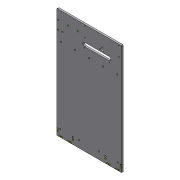
# Autodesk Inventor part: TL20240901-10320CV-002
Saved by Autodesk Inventor 2022.5 (Build 265521000, 521)
## iProperties
Category: FOLLOWER UNIT ASSY
Manager: 호상태
Company: 현대 트랜시스
RuleStatus: InUse
Created: 2023-01-19
Part Number: TL20240901-10320CV-002
Project: MEa-PJT 2LINE
Checked By: 김형민
Engr Approved By: 김형민
User Status: 1/1 x6
Material: SS400
Description: 0
Document SubType Name: Modeling
Mfg Approved By: 호상태
Designer: 박성규
Stock Number: 002
Mass: 13148.3 g
Surface Area: 1560.92 cm^2
Volume: 1670.68 cm^3
Density: 7.85 g/cm^3
Appearance: Painting-RAL7035
BeforeDocSave0: file://Part Design STD iLogic
DETAIL: Coveryor Assembly
M/C TITLE: MEa/NEa차종 시트조립라인
SPECIFICATION: TL20221201-000000CV-005
DocNumber: 221118_Standard_v1
Folder: .\
VDS_Category: 엔지니어링
Detail Description: Processed products
Title: SIDE PLATE
Subject: MEa차종 시트조립2라인
Author: 박성규
Revision Number: A
Autodesk Inventor part; units mm, degrees
ref_plane "YZ Plane" through (0, 0, 0) normal (1, 0, 0) x (0, 1, 0)
ref_plane "XZ Plane" through (0, 0, 0) normal (0, 1, 0) x (-1, 0, 0)
ref_plane "XY Plane" through (0, 0, 0) normal (0, 0, 1) x (1, 0, 0)
sketch "스케치22" plane through (0, 0, 0) normal (0, 0, 1) x (1, 0, 0)
  line L0 (-230, 390) -> (230, 390)
  line L1 (230, 390) -> (230, -390)
  line L2 (230, -390) -> (-230, -390)
  line L3 (-230, -390) -> (-230, 390)
  line L4 (-230, 390) -> (230, -390) construction
  line L5 (230, 390) -> (-230, -390) construction
  point P0 (0, 0)
  dimension "d122" = 460
  dimension "HIGHT" = 780
  constraints: 12 end point, 2 midpoint, 2 parallel, 1 horizontal, 1 perpendicular
  measures "d122" distance of L0.start L0.end
  measures "HIGHT" distance of L0.end L1.end
extrude "돌출12" add sketch "스케치22" along normal blind 12
sketch "스케치23" plane through (0, 0, 12) normal (0, 0, 1) x (1, 0, 0)
  line L0 (230, 390) -> (-230, 390) construction
  line L1 (-230, 390) -> (-230, -390) construction
  point P0 (0, 0)
  point P1 (-220, 324)
  point P2 (-220, 264)
  point P3 (-190, 264)
  point P4 (-150, 324)
  point P5 (-80, 324)
  point P6 (-220, -246)
  point P7 (-150, -246)
  point P8 (-80, -246)
  point P9 (-220, -306)
  point P10 (-190, -306)
  dimension "d126" = 66
  dimension "d128" = 126
  dimension "d129" = 10
  dimension "d130" = 10
  dimension "d131" = 70
  dimension "d132" = 70
  dimension "d133" = 30
  dimension "d154" = 10
  dimension "d155" = 30
  dimension "d156" = 696
  dimension "d157" = 636
  dimension "d158" = 10
  dimension "d159" = 70
  dimension "d160" = 70
  constraints: 6 horizontal alignment
  measures "d126" distance from line of L0 point (-220, 324)
  measures "d128" distance from line of L0 point (-220, 264)
  measures "d129" distance from line of L1 point (-220, 324)
  measures "d130" distance from line of L1 point (-220, 264)
  measures "d131" distance of point (-150, 324) point (-220, 324)
  measures "d132" distance of point (-80, 324) point (-150, 324)
  measures "d133" distance of point (-190, 264) point (-220, 264)
  measures "d154" distance from line of L1 point (-220, -306)
  measures "d155" distance of point (-220, -306) point (-190, -306)
  measures "d156" distance from line of L0 point (-220, -306)
  measures "d157" distance from line of L0 point (-220, -246)
  measures "d158" distance from line of L1 point (-220, -246)
  measures "d159" distance of point (-150, -246) point (-220, -246)
  measures "d160" distance of point (-80, -246) point (-150, -246)
hole "구멍7" at (-220, 324, 12) at (-220, 264, 12) at (-190, 264, 12) at (-150, 324, 12) at (-80, 324, 12) direction (0, 0, -1) diameter 9 end through all clearance for "Socket Head Cap Screw" size "M8" standard "TS Profile"
sketch "스케치24" plane through (0, 0, 12) normal (0, 0, 1) x (1, 0, 0)
  line L0 (230, 390) -> (-230, 390) construction
  line L1 (-230, 390) -> (-230, -390) construction
  line L2 (230, -390) -> (230, 390) construction
  line L3 (-230, -390) -> (230, -390) projected
  point P0 (0, 0)
  point P1 (-200, 198)
  point P2 (-100, 198)
  point P3 (0, 198)
  point P4 (100, 198)
  point P5 (200, 198)
  point P6 (55, -372)
  point P7 (0, -372)
  point P8 (-55, -372)
  point P9 (-110, -372)
  point P10 (110, -372)
  dimension "d141" = 30
  dimension "d142" = 192
  dimension "d143" = 100
  dimension "d144" = 100
  dimension "d145" = 100
  dimension "d146" = 100
  dimension "d231" = 55
  dimension "d234" = 120
  dimension "d308" = 120
  dimension "d338" = 18
  dimension "d339" = 55
  dimension "d340" = 55
  dimension "d341" = 55
  constraints: 8 horizontal alignment
  measures "d141" distance from line of L1 point (-200, 198)
  measures "d142" distance from line of L0 point (-200, 198)
  measures "d143" distance of point (-100, 198) point (-200, 198)
  measures "d144" distance of point (0, 198) point (-100, 198)
  measures "d145" distance of point (0, 198) point (100, 198)
  measures "d146" distance of point (200, 198) point (100, 198)
  measures "d231" distance of point (-55, -372) point (-110, -372)
  measures "d234" distance from line of L1 point (-110, -372)
  measures "d308" distance from line of L2 point (110, -372)
  measures "d338" distance from line of point (-110, -372) L3
  measures "d339" distance of point (0, -372) point (55, -372)
  measures "d340" distance of point (-55, -372) point (0, -372)
  measures "d341" distance of point (55, -372) point (110, -372)
hole "구멍8" at (-200, 198, 12) at (-100, 198, 12) at (0, 198, 12) at (100, 198, 12) at (200, 198, 12) direction (0, 0, -1) diameter 9 end through all clearance for "Socket Head Cap Screw" size "M8" standard "TS Profile"
fillet "모깎기6" radius 5 2 edges at (-230, 390, 6) (230, 390, 6)
sketch "스케치29" plane through (0, 0, 12) normal (0, 0, 1) x (1, 0, 0)
  line L0 (230, -390) -> (230, 385) construction
  line L1 (225, 390) -> (-225, 390) construction
  point P0 (0, 0)
  point P1 (210, 382)
  point P2 (-30, 382)
  point P3 (210, -188)
  point P4 (-30, -188)
  dimension "d199" = 8
  dimension "d200" = 20
  dimension "d201" = 240
  dimension "d202" = 570
  constraints: 2 horizontal alignment, 2 vertical alignment
  measures "d199" distance from line of L1 point (210, 382)
  measures "d200" distance from line of L0 point (210, 382)
  measures "d201" distance of point (-30, 382) point (210, 382)
  measures "d202" distance of point (210, -188) point (210, 382)
hole "구멍11" at (210, 382, 12) at (-30, 382, 12) direction (0, 0, -1) diameter 4.917 end through all thread size "M6x1" class "6H" standard "TS profile"
sketch "스케치31" plane through (0, 0, 0) normal (0, 0, -1) x (-1, 0, 0)
  line L0 (-230, -390) -> (-230, 385) construction
  line L1 (-225, 390) -> (225, 390) construction
  point P0 (-75, 375)
  point P1 (-162, 375)
  point P2 (0, 0)
  point P3 (-210, 311)
  point P4 (-90, 311)
  point P5 (30, 311)
  point P6 (-198, 375)
  point P7 (-196, 375)
  dimension "d219" = 79
  dimension "d220" = 20
  dimension "d221" = 120
  dimension "d222" = 120
  constraints: 2 horizontal alignment, 1 other
  measures "d220" distance from line of L0 point (-210, 311)
  measures "d221" distance of point (-90, 311) point (-210, 311)
  measures "d222" distance of point (-90, 311) point (30, 311)
hole "구멍13" at (210, 311, 0) at (90, 311, 0) at (-30, 311, 0) direction (0, 0, 1) diameter 6.6 end through all clearance for "Socket Head Cap Screw" size "M6" standard "TS Profile"
sketch "스케치43" plane through (0, 0, 0) normal (0, 0, -1) x (-1, 0, 0)
  line L0 (230, 385) -> (230, -390) projected
  line L1 (230, -390) -> (-230, -390) projected
  point P0 (0, 0)
  point P1 (205, -340)
  point P2 (70, -340)
  point P3 (-70, -340)
  point P4 (-205, -340)
  dimension "d309" = 135
  dimension "d310" = 140
  dimension "d311" = 135
  dimension "d312" = 25
  dimension "d314" = 50
  constraints: 3 horizontal alignment
  measures "d309" distance of point (70, -340) point (205, -340)
  measures "d310" distance of point (-70, -340) point (70, -340)
  measures "d311" distance of point (-205, -340) point (-70, -340)
  measures "d312" distance from line of L0 point (205, -340)
  measures "d314" distance from line of L1 point (205, -340)
hole "구멍18" at (-205, -340, 0) at (-70, -340, 0) at (70, -340, 0) at (205, -340, 0) direction (0, 0, 1) diameter 9 end through all clearance for "Socket Head Cap Screw" size "M8" standard "TS Profile"
sketch "스케치44" plane through (0, 0, 12) normal (0, 0, 1) x (1, 0, 0)
  line L0 (-116, -361) -> (-224, -361)
  line L1 (-224, -361) -> (-224, -346)
  line L2 (-224, -346) -> (-116, -346)
  line L3 (-116, -346) -> (-116, -361)
  line L4 (-116, -361) -> (-224, -346) construction
  line L5 (-224, -361) -> (-116, -346) construction
  line L6 (-230, 385) -> (-230, -390) projected
  line L7 (-230, -390) -> (230, -390) projected
  point P0 (0, 0)
  point P1 (-210, -384)
  point P2 (-195, -384)
  point P3 (-145, -384)
  point P4 (-130, -384)
  point P5 (-170, -353.5)
  dimension "d322" = 108
  dimension "d323" = 15
  dimension "d324" = 20
  dimension "d325" = 15
  dimension "d326" = 50
  dimension "d327" = 15
  dimension "d328" = 6
  dimension "d329" = 29
  dimension "d330" = 6
  constraints: 12 end point, 3 horizontal alignment, 2 midpoint, 2 parallel, 1 horizontal, 1 perpendicular
  measures "d322" distance of L0.start L0.end
  measures "d323" distance of L2.end L0.start
  measures "d324" distance from line of L6 point (-210, -384)
  measures "d325" distance of point (-195, -384) point (-210, -384)
  measures "d326" distance of point (-145, -384) point (-195, -384)
  measures "d327" distance of point (-130, -384) point (-145, -384)
  measures "d328" distance between parallel lines of L6 L1
  measures "d329" distance between parallel lines of L7 L0
  measures "d330" distance from line of L7 point (-210, -384)
hole "구멍19" at (-210, -384, 12) at (-195, -384, 12) at (-145, -384, 12) at (-130, -384, 12) at (-224, -361, 12) at (-224, -346, 12) at (-116, -361, 12) at (-116, -346, 12) direction (0, 0, -1) diameter 6.6 end through all counterbore diameter 11 counterbore depth 6.5 clearance for "Socket Head Cap Screw" size "M6" standard "TS Profile"
mirror "미러2" about plane through (0, 0, 0) normal (1, 0, 0) of "구멍19"
sketch "Sketch45" plane through (0, 0, 0) normal (0, 0, -1) x (-1, 0, 0)
  line L0 (-155, 254) -> (45, 254)
  line L1 (45, 254) -> (45, 280)
  line L2 (45, 280) -> (-155, 280)
  line L3 (-155, 280) -> (-155, 254)
  line L4 (-230, -390) -> (-230, 385) projected
  line L5 (-225, 390) -> (225, 390) projected
  point P0 (0, 0)
  dimension "d342" = 200
  dimension "d343" = 26
  dimension "d344" = 75
  dimension "d345" = 110
  constraints: 8 end point, 2 parallel, 1 horizontal, 1 perpendicular
  measures "d342" distance of L2.end L1.end
  measures "d343" distance of L1.end L0.end
  measures "d344" distance between parallel lines of L4 L3
  measures "d345" distance between parallel lines of L5 L2
extrude "Extrusion22" cut sketch "Sketch45" along normal through all both and the other way through all
sketch "Sketch46" plane through (0, 0, 0) normal (0, 0, -1) x (-1, 0, 0)
  line L0 (45, 254) -> (-155, 254) projected
  line L1 (-155, 254) -> (-155, 280) projected
  line L2 (45, 280) -> (45, 254) projected
  point P0 (0, 0)
  point P1 (-145, 244.5)
  point P2 (35, 244.5)
  dimension "d348" = 9.5
  dimension "d349" = 10
  dimension "d350" = 10
  constraints: 1 horizontal alignment
  measures "d348" distance from line of point (-145, 244.5) L0
  measures "d349" distance from line of point (-145, 244.5) L1
  measures "d350" distance from line of point (35, 244.5) L2
hole "Hole20" at (145, 244.5, 0) at (-35, 244.5, 0) direction (0, 0, 1) diameter 4.134 end through all thread size "M5x0.8" class "6H" standard "TS profile"
fillet "Fillet8" radius 13 4 edges at (155, 254, 6) (155, 280, 6) (-45, 254, 6) (-45, 280, 6)
sketch "Sketch47" plane through (0, 0, 0) normal (0, 0, -1) x (-1, 0, 0)
  line L0 (-80, 294.35) -> (-100, 294.35) construction
  line L1 (-80, 299.35) -> (-100, 299.35)
  line L2 (-100, 289.35) -> (-80, 289.35)
  arc A0 (-80, 289.35) -> (-80, 299.35) centre (-80, 294.35) ccw
  arc A1 (-100, 299.35) -> (-100, 289.35) centre (-100, 294.35) ccw
  line L3 (-230, -390) -> (-230, 385) projected
  line L4 (-225, 390) -> (225, 390) projected
  point P0 (0, 0)
  point P1 (-90, 294.35)
  dimension "d359" = 10
  dimension "d360" = 10
  dimension "d361" = 140
  dimension "d362" = 95.65
  constraints: 8 end point, 4 point on circle, 4 tangent, 2 centre point, 1 horizontal, 1 midpoint, 1 parallel
  measures "d359" distance of point (-90, 294.35) L0.end
  measures "d360" diameter of A1
  measures "d361" distance from line of point (-90, 294.35) L3
  measures "d362" distance between parallel lines of L4 L0
extrude "Extrusion23" cut sketch "Sketch47" along normal through all both and the other way through all
equation "\"d132\" = d131"
equation "\"d160\" = d159"
equation "\"d144\" = d143"
equation "\"d145\" = d143"
equation "\"d146\" = d143"
